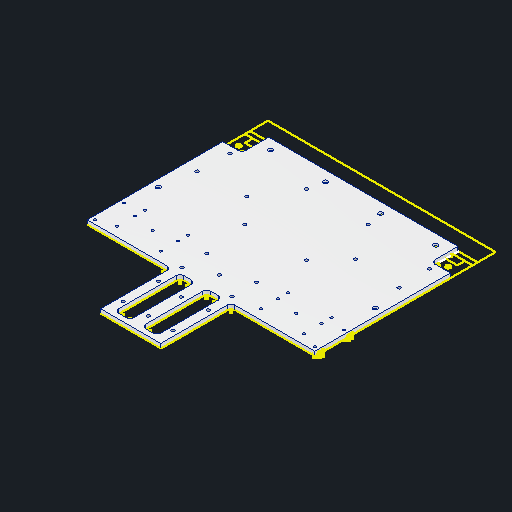
# Autodesk Inventor part: base
Saved by Autodesk Inventor 2023 (Build 270158000, 158)
## iProperties
Created: 2024-04-10
Part Number: base
Material: Aluminum 6061
Document SubType Name: Modeling
Designer: szymo
Density: 2.7 g/cm^3
Appearance: Aluminum - Flat
Mass: 187.188 g
Surface Area: 501.435 cm^2
Volume: 69.3287 cm^3
Author: szymo
Autodesk Inventor part; units mm, degrees
ref_plane "YZ Plane" through (0, 0, 0) normal (1, 0, 0) x (0, 1, 0)
ref_plane "XZ Plane" through (0, 0, 0) normal (0, 1, 0) x (-1, 0, 0)
ref_plane "XY Plane" through (0, 0, 0) normal (0, 0, 1) x (1, 0, 0)
sketch "Sketch2" plane through (0, 0, 0) normal (0, 1, 0) x (-1, 0, 0)
  line L0 (-89, 99) -> (89, 99)
  line L1 (89, 99) -> (89, -99)
  line L2 (89, -99) -> (-89, -99)
  line L3 (-89, -99) -> (-89, 99)
  line L4 (-89, 99) -> (89, -99) construction
  line L5 (89, 99) -> (-89, -99) construction
  line L6 (-89, 99) -> (89, 99)
  line L7 (89, 99) -> (89, -85)
  line L8 (89, -85) -> (-89, -85)
  line L9 (-89, -85) -> (-89, 99)
  line L10 (-4.5, 99) -> (-89, 99)
  line L11 (-89, 99) -> (-89, 42)
  line L12 (-89, 42) -> (-4.5, 42)
  line L13 (-4.5, 42) -> (-4.5, 99)
  line L14 (4.5, 99) -> (89, 99)
  line L15 (89, 99) -> (89, 42)
  line L16 (89, 42) -> (4.5, 42)
  line L17 (4.5, 42) -> (4.5, 99)
  line L18 (22.5, 77.5) -> (22.5, 66.5) projected
  line L19 (16.5, 66.5) -> (16.5, 77.5) projected
  line L20 (-22.5, 66.5) -> (-22.5, 77.5) projected
  line L21 (-16.5, 77.5) -> (-16.5, 66.5) projected
  line L22 (-23.5, 99) -> (-16.5, 99)
  line L23 (-16.5, 99) -> (-16.5, 42)
  line L24 (-16.5, 42) -> (-23.5, 42)
  line L25 (-23.5, 42) -> (-23.5, 99)
  line L26 (16.5, 99) -> (23.5, 99)
  line L27 (23.5, 99) -> (23.5, 42)
  line L28 (23.5, 42) -> (16.5, 42)
  line L29 (16.5, 42) -> (16.5, 99)
  line L30 (-89, 99) -> (89, 99)
  line L31 (89, 99) -> (89, 97)
  line L32 (89, 97) -> (-89, 97)
  line L33 (-89, 97) -> (-89, 99)
  line L34 (89, -85) -> (74, -85)
  line L35 (74, -85) -> (74, -64)
  line L36 (74, -64) -> (89, -64)
  line L37 (89, -64) -> (89, -85)
  line L38 (-89, -85) -> (-74, -85)
  line L39 (-74, -85) -> (-74, -64)
  line L40 (-74, -64) -> (-89, -64)
  line L41 (-89, -64) -> (-89, -85)
  line L42 (16.5, 97) -> (-16.5, 97)
  line L43 (-16.5, 97) -> (-16.5, 93)
  line L44 (-16.5, 93) -> (16.5, 93)
  line L45 (16.5, 93) -> (16.5, 97)
  line L46 (-84.4, -75) -> (-84.4, -71.5) projected
  line L47 (-84.4, -71.5) -> (-87, -71.5) projected
  line L48 (-87, -71.5) -> (-87, -75) projected
  line L49 (-87, -75) -> (-84.4, -75) projected
  line L50 (-79.6, -75) -> (-77, -75) projected
  line L51 (-77, -75) -> (-77, -71.5) projected
  line L52 (-77, -71.5) -> (-79.6, -71.5) projected
  line L53 (-79.6, -71.5) -> (-79.6, -75) projected
  line L54 (-75, -78) -> (-89, -78) projected
  line L55 (-89, -78) -> (-89, -63) projected
  line L56 (-89, -63) -> (-75, -63) projected
  line L57 (-75, -63) -> (-75, -78) projected
  circle A0 centre (-80.45, -67.25) radius 1.25 projected
  point P0 (0, 0)
  point P1 (4.5, 99)
  point P2 (-4.5, 99)
  point P3 (-89, 42)
  point P4 (89, 42)
  point P5 (4.5, 97)
  point P6 (-4.5, 97)
  point P7 (-16.5, 97)
  point P8 (-23.5, 97)
  point P9 (23.5, 97)
  point P10 (16.5, 98)
  point P11 (-4.5, 93)
  point P12 (4.5, 93)
  point P13 (16.5, 93)
  dimension "d8" = 178
  dimension "d9" = 198
  dimension "d10" = 14
  dimension "d11" = 84.5
  dimension "d13" = 84.5
  dimension "d17" = 9
  dimension "d18" = 2
  dimension "d19" = 15
  dimension "d20" = 21
  dimension "d21" = 15
  dimension "d22" = 21
  dimension "d75" = 55
  dimension "d76" = 55
  dimension "d77" = 7
  dimension "d78" = 7
  dimension "d79" = 4
  constraints: 84 end point, 20 parallel, 10 horizontal, 10 perpendicular, 10 point on line, 2 collinear, 2 midpoint, 5 other
  measures "d8" distance of L1.end L2.end
  measures "d9" distance of L0.end L1.end
  measures "d10" distance between parallel lines of L8 L2
  measures "d11" distance of L12.end L11.end
  measures "d13" distance of L15.end L16.end
  measures "d17" distance between parallel lines of L13 L17
  measures "d18" distance of L30.end L31.end
  measures "d19" distance of L35.end L36.end
  measures "d20" distance of L34.end L35.end
  measures "d21" distance of L40.end L39.end
  measures "d22" distance of L39.end L38.end
  measures "d75" distance between parallel lines of L32 L12
  measures "d76" distance between parallel lines of L32 L16
  measures "d77" distance between parallel lines of L23 L25
  measures "d78" distance between parallel lines of L27 L29
  measures "d79" distance of L43.end L42.end
extrude "Extrusion2" add sketch "Sketch2" along normal blind 3 contours L32 L23 L21 L12 L25 | L12 L13 L44 L17 L16 L1 L36 L35 L8 L39 L40 L57 L56 L3 | L32 L13 L44 L23 | L56 L57 L40 L3 | L32 L17 L44 L13 | L32 L29 L44 L17 | L32 L27 L16 L29 L19
fillet "Fillet5" radius 3 12 edges at (-16.5, 1.5, 42) (-4.5, 1.5, 42) (-23.5, 1.5, 42) (16.5, 1.5, 42) (-16.5, 1.5, 93) (-4.5, 1.5, 93) (4.5, 1.5, 93) (16.5, 1.5, 93) (4.5, 1.5, 42) (23.5, 1.5, 42) (74, 1.5, -64) (-74, 1.5, -64)
sketch "Sketch7" plane through (0, 3, 0) normal (0, 1, 0) x (1, 0, 0)
  circle A0 centre (78, 58.6725) radius 1.8 projected
  circle A1 centre (79, 33.8889) radius 1.8 projected
  circle A2 centre (42.4984, 36.1666) radius 1.8 projected
  circle A3 centre (24.1, 64.6) radius 1.6 projected
  circle A4 centre (24.1, 16.4) radius 1.6 projected
  circle A5 centre (-24.1, 16.4) radius 1.6 projected
  circle A6 centre (-24.1, 64.6) radius 1.6 projected
  circle A7 centre (-42.5, 36.1649) radius 1.8 projected
  circle A8 centre (-79, 33.8889) radius 1.8 projected
  circle A9 centre (-78, 58.6725) radius 1.8 projected
  circle A10 centre (19.5, -18.05) radius 1.8 projected
  circle A11 centre (19.5, -37.375) radius 1.8 projected
  circle A12 centre (19.5, -55.8) radius 1.8 projected
  circle A13 centre (19.4231, -83.3077) radius 1.8 projected
  circle A14 centre (0, -83.2) radius 1.8 projected
  circle A15 centre (-19.4231, -83.3077) radius 1.8 projected
  circle A16 centre (-19.5, -55.8) radius 1.8 projected
  circle A17 centre (0, -57.55) radius 1.8 projected
  circle A18 centre (0, -27.625) radius 1.8 projected
  circle A19 centre (-19.5, -37.375) radius 1.8 projected
  circle A20 centre (-19.5, -18.05) radius 1.8 projected
  point P0 (0, 0)
  point P1 (-19.5, -83.2)
  constraints: 20 coincident
hole "Hole3" at (19.4231, 3, 83.3077) at (0, 3, 83.2) at (-19.5, 3, 83.2) at (19.5, 3, 55.8) at (0, 3, 57.55) at (-19.5, 3, 55.8) at (-19.5, 3, 37.375) at (-19.5, 3, 18.05) at (0, 3, 27.625) at (19.5, 3, 37.375) at (19.5, 3, 18.05) at (79, 3, -33.8889) at (78, 3, -58.6725) at (42.4984, 3, -36.1666) at (24.1, 3, -16.4) at (-24.1, 3, -16.4) at (-24.1, 3, -64.6) at (24.1, 3, -64.6) at (-42.5, 3, -36.1649) at (-78, 3, -58.6725) at (-79, 3, -33.8889) direction (0, -1, 0) diameter 2.459 end through all thread size "M3x0.5" class "6H" standard "ISO Metric profile"
sketch "Sketch8" plane through (0, 3, 0) normal (0, 1, 0) x (1, 0, 0)
  circle A0 centre (72.95, -34.475) radius 1.45 projected
  circle A1 centre (72.95, -20.775) radius 1.45 projected
  circle A2 centre (39.125, -20.8375) radius 1.55 projected
  circle A3 centre (39.125, -34.4125) radius 1.55 projected
  circle A4 centre (-39.125, -20.8375) radius 1.55 projected
  circle A5 centre (-39.125, -34.4125) radius 1.55 projected
  circle A6 centre (-72.95, -34.475) radius 1.45 projected
  circle A7 centre (-72.95, -20.775) radius 1.45 projected
  circle A8 centre (86, -16.25) radius 2.3 projected
  circle A9 centre (86, -39) radius 2.3 projected
  circle A10 centre (86, 32.8889) radius 2.3 projected
  line L0 (89, -42) -> (83, -42) projected
  line L1 (89, 35.8889) -> (89, -42) projected
  line L2 (89, 35.8889) -> (83, 35.8889) projected
  line L3 (83, 29.8889) -> (83, 35.8889) projected
  line L4 (83, 29.8889) -> (87.4, 29.8889) projected
  line L5 (87.4, 29.8889) -> (87.4, 14.7889) projected
  line L6 (87.4, 14.7889) -> (79.4, 14.7889) projected
  line L7 (79.4, 2.7889) -> (79.4, 14.7889) projected
  line L8 (86, 2.7889) -> (79.4, 2.7889) projected
  line L9 (86, -13.25) -> (86, 2.7889) projected
  line L10 (86, -13.25) -> (83, -13.25) projected
  line L11 (83, -13.25) -> (83, -19.25) projected
  line L12 (83, -19.25) -> (86, -19.25) projected
  line L13 (86, -36) -> (86, -19.25) projected
  line L14 (86, -36) -> (83, -36) projected
  line L15 (83, -36) -> (83, -42) projected
  circle A11 centre (83.4, 10.7889) radius 2.6 projected
  circle A12 centre (-86, -39) radius 2.3 projected
  circle A13 centre (-86, -16.25) radius 2.3 projected
  line L16 (-86, -13.25) -> (-86, -0.1111) projected
  line L17 (-79.4, -0.1111) -> (-86, -0.1111) projected
  line L18 (-79.4, 11.8889) -> (-79.4, -0.1111) projected
  line L19 (-86, 11.8889) -> (-79.4, 11.8889) projected
  line L20 (-86, 11.8889) -> (-86, 29.8889) projected
  line L21 (-86, 29.8889) -> (-83, 29.8889) projected
  line L22 (-83, 29.8889) -> (-83, 35.8889) projected
  line L23 (-89, 35.8889) -> (-83, 35.8889) projected
  line L24 (-89, 35.8889) -> (-89, -42) projected
  line L25 (-89, -42) -> (-83, -42) projected
  line L26 (-83, -42) -> (-83, -36) projected
  line L27 (-83, -36) -> (-86, -36) projected
  line L28 (-86, -36) -> (-86, -19.25) projected
  line L29 (-86, -19.25) -> (-83, -19.25) projected
  line L30 (-83, -19.25) -> (-83, -13.25) projected
  line L31 (-83, -13.25) -> (-86, -13.25) projected
  circle A14 centre (-86, 32.8889) radius 2.3 projected
  circle A15 centre (-83.4, 7.8889) radius 2.6 projected
  line L32 (72.95, -34.475) -> (39.125, -12.8375)
  line L33 (72.95, -12.775) -> (39.125, -34.4125)
  line L34 (-39.125, -34.4125) -> (-72.95, -12.775)
  line L35 (-39.125, -12.8375) -> (-72.95, -34.4125)
  point P0 (0, 0)
  point P1 (56.0375, -23.5937)
  point P2 (-56.0375, -23.625)
  dimension "d90" = 8
  dimension "d91" = 8
  dimension "d92" = 8
  dimension "d93" = 8
  constraints: 12 coincident, 8 end point, 2 midpoint
  measures "d90" distance of A1.centre L33.start
  measures "d91" distance of L32.end A2.centre
  measures "d92" distance of point (-39.125, -20.837) L35.start
  measures "d93" distance of A7.centre L34.end
hole "Hole4" at (72.95, 3, 34.475) at (72.95, 3, 20.775) at (39.125, 3, 20.8375) at (39.125, 3, 34.4125) at (86, 3, 39) at (86, 3, 16.25) at (-86, 3, 39) at (-86, 3, 16.25) at (-72.95, 3, 20.775) at (-72.95, 3, 34.475) at (-39.125, 3, 34.4125) at (-39.125, 3, 20.8375) at (72.95, 3, 12.775) at (39.125, 3, 12.8375) at (-39.125, 3, 12.8375) at (-72.95, 3, 12.775) at (56.0375, 3, 23.5937) at (-56.0375, 3, 23.625) direction (0, -1, 0) diameter 2.013 end through all thread size "M2.5x0.45" class "6H" standard "ISO Metric profile"
sketch "Sketch9" plane through (0, 0, 0) normal (0, -1, 0) x (1, 0, 0)
  circle A0 centre (64.5, -77) radius 1.2295 projected
  circle A1 centre (21.5, -77) radius 1.2295 projected
  circle A2 centre (-21.5, -77) radius 1.2295 projected
  circle A3 centre (-64.5, -77) radius 1.2295 projected
  circle A4 centre (-83.4, -7.8889) radius 2.6 projected
  circle A5 centre (83.4, -10.7889) radius 2.6 projected
  point P0 (0, 0)
  constraints: 6 coincident
hole "Hole5" at (-83.4, 0, -7.8889) at (83.4, 0, -10.7889) at (64.5, 0, -77) at (21.5, 0, -77) at (-21.5, 0, -77) at (-64.5, 0, -77) direction (0, 1, 0) diameter 3.6 end through all countersink diameter 6.6 countersink angle 90 clearance for "Countersunk Flat Head Screw ISO 2009/7046" size "M3" standard "ISO"
sketch "Sketch11" plane through (0, 0, 0) normal (0, -1, 0) x (1, 0, 0)
  circle A0 centre (-21.5, -77) radius 3.3 projected
  circle A1 centre (64.5, -77) radius 3.3 projected
  circle A2 centre (-83.4, -7.8889) radius 3.3 projected
  circle A3 centre (83.4, -10.7889) radius 3.3 projected
  circle A4 centre (21.5, -77) radius 3.3 projected
  circle A5 centre (-64.5, -77) radius 3.3 projected
  circle A6 centre (56.0375, 23.5937) radius 1.0065 projected
  circle A7 centre (-39.125, 12.8375) radius 1.0065 projected
  circle A8 centre (72.95, 12.775) radius 1.0065 projected
  circle A9 centre (-39.125, 34.4125) radius 1.0065 projected
  circle A10 centre (-72.95, 20.775) radius 1.0065 projected
  circle A11 centre (-86, 39) radius 1.0065 projected
  circle A12 centre (86, 39) radius 1.0065 projected
  circle A13 centre (39.125, 20.8375) radius 1.0065 projected
  circle A14 centre (72.95, 34.475) radius 1.0065 projected
  circle A15 centre (72.95, 20.775) radius 1.0065 projected
  circle A16 centre (39.125, 34.4125) radius 1.0065 projected
  circle A17 centre (86, 16.25) radius 1.0065 projected
  circle A18 centre (-86, 16.25) radius 1.0065 projected
  circle A19 centre (-72.95, 34.475) radius 1.0065 projected
  circle A20 centre (-39.125, 20.8375) radius 1.0065 projected
  circle A21 centre (39.125, 12.8375) radius 1.0065 projected
  circle A22 centre (-72.95, 12.775) radius 1.0065 projected
  circle A23 centre (-56.0375, 23.625) radius 1.0065 projected
  circle A24 centre (-78, -58.6725) radius 1.2295 projected
  circle A25 centre (24.1, -64.6) radius 1.2295 projected
  circle A26 centre (-24.1, -16.4) radius 1.2295 projected
  circle A27 centre (42.4984, -36.1666) radius 1.2295 projected
  circle A28 centre (79, -33.8889) radius 1.2295 projected
  circle A29 centre (19.5, 37.375) radius 1.2295 projected
  circle A30 centre (-19.5, 18.05) radius 1.2295 projected
  circle A31 centre (-19.5, 55.8) radius 1.2295 projected
  circle A32 centre (19.5, 55.8) radius 1.2295 projected
  circle A33 centre (0, 83.2) radius 1.2295 projected
  circle A34 centre (19.4231, 83.3077) radius 1.2295 projected
  circle A35 centre (-19.5, 83.2) radius 1.2295 projected
  circle A36 centre (0, 57.55) radius 1.2295 projected
  circle A37 centre (-19.5, 37.375) radius 1.2295 projected
  circle A38 centre (0, 27.625) radius 1.2295 projected
  circle A39 centre (19.5, 18.05) radius 1.2295 projected
  circle A40 centre (78, -58.6725) radius 1.2295 projected
  circle A41 centre (24.1, -16.4) radius 1.2295 projected
  circle A42 centre (-24.1, -64.6) radius 1.2295 projected
  circle A43 centre (-42.5, -36.1649) radius 1.2295 projected
  circle A44 centre (-79, -33.8889) radius 1.2295 projected
  arc A45 (-13.5, 93) -> (-16.5, 90) centre (-13.5, 90) ccw projected
  line L0 (-7.5, 93) -> (-13.5, 93) projected
  arc A46 (-4.5, 90) -> (-7.5, 93) centre (-7.5, 90) ccw projected
  line L1 (-4.5, 45) -> (-4.5, 90) projected
  arc A47 (-7.5, 42) -> (-4.5, 45) centre (-7.5, 45) ccw projected
  line L2 (-13.5, 42) -> (-7.5, 42) projected
  arc A48 (-16.5, 45) -> (-13.5, 42) centre (-13.5, 45) ccw projected
  line L3 (-16.5, 90) -> (-16.5, 45) projected
  arc A49 (16.5, 90) -> (13.5, 93) centre (13.5, 90) ccw projected
  line L4 (16.5, 45) -> (16.5, 90) projected
  arc A50 (13.5, 42) -> (16.5, 45) centre (13.5, 45) ccw projected
  line L5 (7.5, 42) -> (13.5, 42) projected
  arc A51 (4.5, 45) -> (7.5, 42) centre (7.5, 45) ccw projected
  line L6 (4.5, 90) -> (4.5, 45) projected
  arc A52 (7.5, 93) -> (4.5, 90) centre (7.5, 90) ccw projected
  line L7 (13.5, 93) -> (7.5, 93) projected
  line L8 (-23.5, 97) -> (23.5, 97) projected
  line L9 (-23.5, 45) -> (-23.5, 97) projected
  arc A53 (-26.5, 42) -> (-23.5, 45) centre (-26.5, 45) ccw projected
  line L10 (-89, 42) -> (-26.5, 42) projected
  line L11 (-89, -64) -> (-89, 42) projected
  line L12 (-77, -64) -> (-89, -64) projected
  arc A54 (-74, -67) -> (-77, -64) centre (-77, -67) ccw projected
  line L13 (-74, -85) -> (-74, -67) projected
  line L14 (74, -85) -> (-74, -85) projected
  line L15 (74, -67) -> (74, -85) projected
  arc A55 (77, -64) -> (74, -67) centre (77, -67) ccw projected
  line L16 (89, -64) -> (77, -64) projected
  line L17 (89, 42) -> (89, -64) projected
  line L18 (26.5, 42) -> (89, 42) projected
  arc A56 (23.5, 45) -> (26.5, 42) centre (26.5, 45) ccw projected
  line L19 (23.5, 97) -> (23.5, 45) projected
  circle A57 centre (-42.5, -36.1649) radius 1.8 projected
  line L20 (-86, 0.1111) -> (-86, 42) projected
  line L21 (-89, 42) -> (-86, 42) projected
  line L22 (-89, 42) -> (-89, 38.75) projected
  line L23 (-89, 38.75) -> (-89, 13.5) projected
  line L24 (-89, 13.5) -> (-89, -81) projected
  line L25 (-89, -81) -> (-83, -81) projected
  line L26 (-83, -81) -> (-83, -75) projected
  line L27 (-83, -75) -> (-73, -75) projected
  line L28 (-73, -75) -> (-73, -53.3451) projected
  line L29 (-73, -53.3451) -> (-67, -53.3451) projected
  line L30 (-67, -53.3451) -> (-67, -42.9318) projected
  line L31 (-76.801, -42.9318) -> (-67, -42.9318) projected
  ellipse E0 centre (-76.799, -27.2986) end of major axis (-76.7969, -11.6653) minor radius 1.851 (-77.5308, -41.6649) -> (-76.801, -42.9318) ccw projected
  line L32 (-46, -41.6649) -> (-77.5308, -41.6649) projected
  line L33 (-46, -39.6649) -> (-46, -41.6649) projected
  line L34 (-39, -39.6649) -> (-46, -39.6649) projected
  line L35 (-39, -32.6649) -> (-39, -39.6649) projected
  line L36 (-46, -32.6649) -> (-39, -32.6649) projected
  line L37 (-52, -34.8889) -> (-52, -29.8889) projected
  line L38 (-75, -34.8889) -> (-52, -34.8889) projected
  line L39 (-75, -34.8889) -> (-75, -29.8889) projected
  line L40 (-86, -29.8889) -> (-75, -29.8889) projected
  line L41 (-86, -29.8889) -> (-86, -11.8889) projected
  line L42 (-79.4, -11.8889) -> (-86, -11.8889) projected
  line L43 (-79.4, 0.1111) -> (-79.4, -11.8889) projected
  line L44 (-86, 0.1111) -> (-79.4, 0.1111) projected
  circle A58 centre (-83.5, -70.5) radius 1.75 projected
  circle A59 centre (-79, -33.8889) radius 1.8 projected
  circle A60 centre (-83.4, -7.8889) radius 2.6 projected
  circle A61 centre (-78, -58.6725) radius 1.8 projected
  circle A62 centre (78, -58.6725) radius 1.8 projected
  circle A63 centre (79, -33.8889) radius 1.8 projected
  circle A64 centre (83.4, -10.7889) radius 2.6 projected
  circle A65 centre (80.5, -70.5) radius 1.75 projected
  circle A66 centre (42.4984, -36.1666) radius 1.8 projected
  spline S0 degree 2 poles (89, 38.051) (88.5208, 39.25) (89, 40.449) knots 0 0 0 0.244949 0.244949 0.244949 weights 1 1.090909 1 projected
  line L45 (89, 42) -> (89, 40.449) projected
  line L46 (89, 42) -> (86, 42) projected
  line L47 (86, -2.7889) -> (86, 42) projected
  line L48 (79.4, -2.7889) -> (86, -2.7889) projected
  line L49 (79.4, -14.7889) -> (79.4, -2.7889) projected
  line L50 (86, -14.7889) -> (79.4, -14.7889) projected
  line L51 (86, -16.7889) -> (86, -14.7889) projected
  line L52 (86, -27.8889) -> (86, -16.7889) projected
  line L53 (86, -29.8889) -> (86, -27.8889) projected
  line L54 (39, -32.6649) -> (46, -32.6649) projected
  line L55 (39, -39.6649) -> (39, -32.6649) projected
  line L56 (46, -39.6649) -> (39, -39.6649) projected
  line L57 (46, -41.6649) -> (46, -39.6649) projected
  line L58 (46, -41.6649) -> (77.5308, -41.6649) projected
  ellipse E1 centre (76.799, -27.2986) end of major axis (76.7969, -11.6653) minor radius 1.851 (76.801, -42.9318) -> (77.5308, -41.6649) ccw projected
  line L59 (76.801, -42.9318) -> (67, -42.9318) projected
  line L60 (67, -53.3451) -> (67, -42.9318) projected
  line L61 (73, -53.3451) -> (67, -53.3451) projected
  line L62 (73, -75) -> (73, -53.3451) projected
  line L63 (83, -75) -> (73, -75) projected
  line L64 (83, -81) -> (83, -75) projected
  line L65 (89, -81) -> (83, -81) projected
  line L66 (89, 14.801) -> (89, -81) projected
  spline S1 degree 2 poles (89, 14.801) (88.5208, 16) (89, 17.199) knots 0 0 0 0.244949 0.244949 0.244949 weights 1 1.090909 1 projected
  line L67 (89, 38.051) -> (89, 17.199) projected
  line L68 (27.5, -68) -> (27.5, -13) projected
  line L69 (27.5, -13) -> (-27.5, -13) projected
  line L70 (-27.5, -13) -> (-27.5, -68) projected
  line L71 (-27.5, -68) -> (27.5, -68) projected
  circle A67 centre (26.5, -56.73) radius 0.325 projected
  circle A68 centre (26.5, -53) radius 0.325 projected
  circle A69 centre (26.5, -54.27) radius 0.325 projected
  circle A70 centre (26.5, -60.54) radius 0.325 projected
  circle A71 centre (24.1, -64.6) radius 1.6 projected
  circle A72 centre (26.5, -58) radius 0.325 projected
  circle A73 centre (26.5, -59.27) radius 0.325 projected
  circle A74 centre (26.5, -50.46) radius 0.325 projected
  circle A75 centre (26.5, -51.73) radius 0.325 projected
  circle A76 centre (24.1, -16.4) radius 1.6 projected
  circle A77 centre (15, -15) radius 0.35 projected
  circle A78 centre (15, -17.5) radius 0.35 projected
  circle A79 centre (7.75, -17.5) radius 0.35 projected
  circle A80 centre (7.75, -15) radius 0.35 projected
  circle A81 centre (0.5, -17.5) radius 0.35 projected
  circle A82 centre (-24.1, -64.6) radius 1.6 projected
  circle A83 centre (-26.5, -59.27) radius 0.325 projected
  circle A84 centre (-26.5, -60.54) radius 0.325 projected
  circle A85 centre (-26.5, -56.73) radius 0.325 projected
  circle A86 centre (-26.5, -58) radius 0.325 projected
  circle A87 centre (-26.5, -53) radius 0.325 projected
  circle A88 centre (-26.5, -54.27) radius 0.325 projected
  circle A89 centre (-6.75, -17.5) radius 0.35 projected
  circle A90 centre (-14, -17.5) radius 0.35 projected
  circle A91 centre (0.5, -15) radius 0.35 projected
  circle A92 centre (-6.75, -15) radius 0.35 projected
  circle A93 centre (-26.5, -50.46) radius 0.325 projected
  circle A94 centre (-26.5, -51.73) radius 0.325 projected
  circle A95 centre (-14, -15) radius 0.35 projected
  circle A96 centre (-24.1, -16.4) radius 1.6 projected
  circle A97 centre (21.5, -77) radius 1.2295 projected
  circle A98 centre (-64.5, -77) radius 1.2295 projected
  circle A99 centre (-21.5, -77) radius 1.2295 projected
  circle A100 centre (64.5, -77) radius 1.2295 projected
  line L72 (-72, -70) -> (-72, -79) projected
  arc A101 (-74, -81) -> (-72, -79) centre (-74, -79) ccw projected
  line L73 (-74, -81) -> (-89, -81) projected
  line L74 (-89, -81) -> (-89, -85) projected
  line L75 (-89, -85) -> (89, -85) projected
  line L76 (89, -81) -> (89, -85) projected
  line L77 (89, -81) -> (74, -81) projected
  arc A102 (72, -79) -> (74, -81) centre (74, -79) ccw projected
  line L78 (72, -79) -> (72, -70) projected
  line L79 (57, -70) -> (72, -70) projected
  line L80 (57, -70) -> (57, -79) projected
  arc A103 (55, -81) -> (57, -79) centre (55, -79) ccw projected
  line L81 (55, -81) -> (31, -81) projected
  arc A104 (29, -79) -> (31, -81) centre (31, -79) ccw projected
  line L82 (29, -79) -> (29, -70) projected
  line L83 (14, -70) -> (29, -70) projected
  line L84 (14, -70) -> (14, -79) projected
  arc A105 (12, -81) -> (14, -79) centre (12, -79) ccw projected
  line L85 (12, -81) -> (-12, -81) projected
  arc A106 (-14, -79) -> (-12, -81) centre (-12, -79) ccw projected
  line L86 (-14, -79) -> (-14, -70) projected
  line L87 (-29, -70) -> (-14, -70) projected
  line L88 (-29, -70) -> (-29, -79) projected
  arc A107 (-31, -81) -> (-29, -79) centre (-31, -79) ccw projected
  line L89 (-31, -81) -> (-55, -81) projected
  arc A108 (-57, -79) -> (-55, -81) centre (-55, -79) ccw projected
  line L90 (-57, -79) -> (-57, -70) projected
  line L91 (-72, -70) -> (-57, -70) projected
  line L92 (-89, -85) -> (-89, -99) projected
  line L93 (-89, -99) -> (89, -99) projected
  line L94 (89, -85) -> (89, -99) projected
  line L95 (-89, -85) -> (89, -85) projected
  circle A109 centre (72.95, 34.475) radius 1.45 projected
  circle A110 centre (72.95, 20.775) radius 1.45 projected
  circle A111 centre (39.125, 34.4125) radius 1.55 projected
  circle A112 centre (39.125, 20.8375) radius 1.55 projected
  spline S2 degree 3 poles (65.7, 23.025) (65.7, 22.8819) (65.6837, 22.6312) (65.6334, 22.3458) (65.5819, 22.1333) (65.5405, 21.9923) (65.48, 21.8179) (65.4239, 21.6792) (65.3456, 21.5106) (65.2769, 21.3802) (65.184, 21.2227) (65.1043, 21.1011) (64.9982, 20.9549) (64.9083, 20.8425) (64.7662, 20.6811) (64.615, 20.5299) (64.3941, 20.3423) (64.2146, 20.2128) (64.0241, 20.0935) (63.8917, 20.0193) (63.7367, 19.9424) (63.63, 19.8951) (63.5206, 19.8513) (63.4473, 19.8241) (63.3368, 19.7865) (63.2255, 19.7528) (63.02, 19.6999) (62.7939, 19.6576) (62.4526, 19.6224) (62.1474, 19.6224) (61.8061, 19.6576) (61.58, 19.6999) (61.3745, 19.7528) (61.2632, 19.7865) (61.1527, 19.8241) (61.0794, 19.8513) (60.97, 19.8951) (60.8633, 19.9424) (60.7083, 20.0193) (60.5759, 20.0935) (60.3854, 20.2128) (60.2059, 20.3423) (59.985, 20.5299) (59.8338, 20.6811) (59.6917, 20.8425) (59.6018, 20.9549) (59.4957, 21.1011) (59.416, 21.2227) (59.3231, 21.3802) (59.2544, 21.5106) (59.1761, 21.6792) (59.12, 21.8179) (59.0595, 21.9923) (59.0181, 22.1333) (58.9666, 22.3458) (58.9163, 22.6312) (58.9, 22.8819) (58.9, 23.025) knots 0.368505 0.368505 0.368505 0.368505 0.400174 0.423925 0.431842 0.447677 0.455594 0.471428 0.479345 0.49518 0.503097 0.518931 0.526849 0.542683 0.5506 0.574352 0.590186 0.613938 0.621855 0.637689 0.645607 0.657482 0.661441 0.669358 0.673317 0.685193 0.69311 0.716861 0.732696 0.764365 0.780199 0.803951 0.811868 0.823744 0.827702 0.835619 0.839578 0.851454 0.859371 0.875205 0.883123 0.906874 0.922709 0.94646 0.954377 0.970212 0.978129 0.993963 1.00188 1.017715 1.025632 1.041466 1.049384 1.065218 1.073135 1.096887 1.128556 1.128556 1.128556 1.128556 projected
  line L96 (58.9, 23.025) -> (58.9, 32.225) projected
  spline S3 degree 3 poles (58.9, 32.225) (58.9, 32.3681) (58.9163, 32.6188) (58.9666, 32.9042) (59.0181, 33.1167) (59.0595, 33.2577) (59.12, 33.4321) (59.1761, 33.5708) (59.2544, 33.7394) (59.3231, 33.8698) (59.416, 34.0273) (59.4957, 34.1489) (59.6018, 34.2951) (59.6917, 34.4075) (59.8338, 34.5689) (59.985, 34.7201) (60.2059, 34.9077) (60.3854, 35.0372) (60.5759, 35.1565) (60.7083, 35.2307) (60.8633, 35.3076) (60.97, 35.3549) (61.0794, 35.3987) (61.1527, 35.4259) (61.2632, 35.4635) (61.3745, 35.4972) (61.58, 35.5501) (61.8061, 35.5924) (62.1474, 35.6276) (62.4526, 35.6276) (62.7939, 35.5924) (63.02, 35.5501) (63.2255, 35.4972) (63.3368, 35.4635) (63.4473, 35.4259) (63.5206, 35.3987) (63.63, 35.3549) (63.7367, 35.3076) (63.8917, 35.2307) (64.0241, 35.1565) (64.2146, 35.0372) (64.3941, 34.9077) (64.615, 34.7201) (64.7662, 34.5689) (64.9083, 34.4075) (64.9982, 34.2951) (65.1043, 34.1489) (65.184, 34.0273) (65.2769, 33.8698) (65.3456, 33.7394) (65.4239, 33.5708) (65.48, 33.4321) (65.5405, 33.2577) (65.5819, 33.1167) (65.6334, 32.9042) (65.6837, 32.6188) (65.7, 32.3681) (65.7, 32.225) knots -0.380025 -0.380025 -0.380025 -0.380025 -0.348357 -0.324605 -0.316688 -0.300853 -0.292936 -0.277102 -0.269185 -0.25335 -0.245433 -0.229599 -0.221682 -0.205847 -0.19793 -0.174178 -0.158344 -0.134592 -0.126675 -0.110841 -0.102924 -0.091048 -0.087089 -0.079172 -0.075213 -0.063338 -0.05542 -0.031669 -0.015834 0.015834 0.031669 0.05542 0.063338 0.075213 0.079172 0.087089 0.091048 0.102924 0.110841 0.126675 0.134592 0.158344 0.174178 0.19793 0.205847 0.221682 0.229599 0.245433 0.25335 0.269185 0.277102 0.292936 0.300853 0.316688 0.324605 0.348357 0.380025 0.380025 0.380025 0.380025 projected
  line L97 (65.7, 32.225) -> (65.7, 23.025) projected
  line L98 (27.2, 42) -> (86, 42) projected
  line L99 (27.2, 13.25) -> (27.2, 42) projected
  line L100 (27.2, 13.25) -> (86, 13.25) projected
  line L101 (86, 42) -> (86, 13.25) projected
  circle A113 centre (-72.95, 34.475) radius 1.45 projected
  circle A114 centre (-72.95, 20.775) radius 1.45 projected
  circle A115 centre (-39.125, 34.4125) radius 1.55 projected
  circle A116 centre (-39.125, 20.8375) radius 1.55 projected
  spline S4 degree 3 poles (-65.7, 23.025) (-65.7, 22.8819) (-65.6837, 22.6312) (-65.6334, 22.3458) (-65.5819, 22.1333) (-65.5405, 21.9923) (-65.48, 21.8179) (-65.4239, 21.6792) (-65.3456, 21.5106) (-65.2769, 21.3802) (-65.184, 21.2227) (-65.1043, 21.1011) (-64.9982, 20.9549) (-64.9083, 20.8425) (-64.7662, 20.6811) (-64.615, 20.5299) (-64.3941, 20.3423) (-64.2146, 20.2128) (-64.0241, 20.0935) (-63.8917, 20.0193) (-63.7367, 19.9424) (-63.63, 19.8951) (-63.5206, 19.8513) (-63.4473, 19.8241) (-63.3368, 19.7865) (-63.2255, 19.7528) (-63.02, 19.6999) (-62.7939, 19.6576) (-62.4526, 19.6224) (-62.1474, 19.6224) (-61.8061, 19.6576) (-61.58, 19.6999) (-61.3745, 19.7528) (-61.2632, 19.7865) (-61.1527, 19.8241) (-61.0794, 19.8513) (-60.97, 19.8951) (-60.8633, 19.9424) (-60.7083, 20.0193) (-60.5759, 20.0935) (-60.3854, 20.2128) (-60.2059, 20.3423) (-59.985, 20.5299) (-59.8338, 20.6811) (-59.6917, 20.8425) (-59.6018, 20.9549) (-59.4957, 21.1011) (-59.416, 21.2227) (-59.3231, 21.3802) (-59.2544, 21.5106) (-59.1761, 21.6792) (-59.12, 21.8179) (-59.0595, 21.9923) (-59.0181, 22.1333) (-58.9666, 22.3458) (-58.9163, 22.6312) (-58.9, 22.8819) (-58.9, 23.025) knots 0.368505 0.368505 0.368505 0.368505 0.400174 0.423925 0.431842 0.447677 0.455594 0.471428 0.479345 0.49518 0.503097 0.518931 0.526849 0.542683 0.5506 0.574352 0.590186 0.613938 0.621855 0.637689 0.645607 0.657482 0.661441 0.669358 0.673317 0.685193 0.69311 0.716861 0.732696 0.764365 0.780199 0.803951 0.811868 0.823744 0.827702 0.835619 0.839578 0.851454 0.859371 0.875205 0.883123 0.906874 0.922709 0.94646 0.954377 0.970212 0.978129 0.993963 1.00188 1.017715 1.025632 1.041466 1.049384 1.065218 1.073135 1.096887 1.128556 1.128556 1.128556 1.128556 projected
  line L102 (-65.7, 32.225) -> (-65.7, 23.025) projected
  spline S5 degree 3 poles (-58.9, 32.225) (-58.9, 32.3681) (-58.9163, 32.6188) (-58.9666, 32.9042) (-59.0181, 33.1167) (-59.0595, 33.2577) (-59.12, 33.4321) (-59.1761, 33.5708) (-59.2544, 33.7394) (-59.3231, 33.8698) (-59.416, 34.0273) (-59.4957, 34.1489) (-59.6018, 34.2951) (-59.6917, 34.4075) (-59.8338, 34.5689) (-59.985, 34.7201) (-60.2059, 34.9077) (-60.3854, 35.0372) (-60.5759, 35.1565) (-60.7083, 35.2307) (-60.8633, 35.3076) (-60.97, 35.3549) (-61.0794, 35.3987) (-61.1527, 35.4259) (-61.2632, 35.4635) (-61.3745, 35.4972) (-61.58, 35.5501) (-61.8061, 35.5924) (-62.1474, 35.6276) (-62.4526, 35.6276) (-62.7939, 35.5924) (-63.02, 35.5501) (-63.2255, 35.4972) (-63.3368, 35.4635) (-63.4473, 35.4259) (-63.5206, 35.3987) (-63.63, 35.3549) (-63.7367, 35.3076) (-63.8917, 35.2307) (-64.0241, 35.1565) (-64.2146, 35.0372) (-64.3941, 34.9077) (-64.615, 34.7201) (-64.7662, 34.5689) (-64.9083, 34.4075) (-64.9982, 34.2951) (-65.1043, 34.1489) (-65.184, 34.0273) (-65.2769, 33.8698) (-65.3456, 33.7394) (-65.4239, 33.5708) (-65.48, 33.4321) (-65.5405, 33.2577) (-65.5819, 33.1167) (-65.6334, 32.9042) (-65.6837, 32.6188) (-65.7, 32.3681) (-65.7, 32.225) knots -0.380025 -0.380025 -0.380025 -0.380025 -0.348357 -0.324605 -0.316688 -0.300853 -0.292936 -0.277102 -0.269185 -0.25335 -0.245433 -0.229599 -0.221682 -0.205847 -0.19793 -0.174178 -0.158344 -0.134592 -0.126675 -0.110841 -0.102924 -0.091048 -0.087089 -0.079172 -0.075213 -0.063338 -0.05542 -0.031669 -0.015834 0.015834 0.031669 0.05542 0.063338 0.075213 0.079172 0.087089 0.091048 0.102924 0.110841 0.126675 0.134592 0.158344 0.174178 0.19793 0.205847 0.221682 0.229599 0.245433 0.25335 0.269185 0.277102 0.292936 0.300853 0.316688 0.324605 0.348357 0.380025 0.380025 0.380025 0.380025 projected
  line L103 (-58.9, 23.025) -> (-58.9, 32.225) projected
  line L104 (-27.2, 42) -> (-86, 42) projected
  line L105 (-86, 42) -> (-86, 13.25) projected
  line L106 (-27.2, 13.25) -> (-86, 13.25) projected
  line L107 (-27.2, 13.25) -> (-27.2, 42) projected
  line L108 (-22.5, 14.25) -> (22.5, 14.25) projected
  line L109 (22.5, 14.25) -> (22.5, 13.25) projected
  line L110 (-22.5, 13.25) -> (22.5, 13.25) projected
  line L111 (-22.5, 14.25) -> (-22.5, 13.25) projected
  line L112 (-27.2, 13.25) -> (-27.2, 42) projected
  line L113 (-27.2, 13.25) -> (-22.7, 13.25) projected
  line L114 (-22.7, 13.25) -> (-22.7, 42) projected
  line L115 (-27.2, 42) -> (-22.7, 42) projected
  line L116 (27.2, 13.25) -> (27.2, 42) projected
  line L117 (27.2, 42) -> (22.7, 42) projected
  line L118 (22.7, 13.25) -> (22.7, 42) projected
  line L119 (27.2, 13.25) -> (22.7, 13.25) projected
  line L120 (-77.0142, -3.75) -> (-9.0142, -3.75) projected
  line L121 (-9.0142, -3.75) -> (-9.0142, 11.25) projected
  line L122 (-9.0142, 11.25) -> (-77.0142, 11.25) projected
  line L123 (-77.0142, 11.25) -> (-77.0142, -3.75) projected
  line L124 (77.6433, -8.75) -> (11.6433, -8.75) projected
  line L125 (77.6433, 11.25) -> (77.6433, -8.75) projected
  line L126 (11.6433, 11.25) -> (77.6433, 11.25) projected
  line L127 (11.6433, -8.75) -> (11.6433, 11.25) projected
  line L128 (-74, -85) -> (74, -85)
  line L129 (74, -85) -> (74, -70)
  line L130 (74, -70) -> (-74, -70)
  line L131 (-74, -70) -> (-74, -85)
  line L132 (86, -29.8889) -> (46, -29.8889) projected
  line L133 (46, -32.6649) -> (46, -29.8889) projected
  line L134 (-46, -29.8889) -> (-46, -32.6649) projected
  line L135 (-46, -29.8889) -> (-52, -29.8889) projected
  point P0 (0, 0)
  constraints: 8 end point, 2 parallel, 1 collinear, 1 horizontal, 1 perpendicular, 1 point on line, 2 other
equation "\"d11\" = d13"
body "Solid2"
